Autodesk Fusion 360 part; units mm, degrees
note: some values were not read from the file. Set by a fixed rule: which face or edge a step refers to; which sketch regions a step uses.
(part 2 of 2)
sketch "Sketch3 (3)" plane through (0, 0, 1.5) normal (0, 0, -1) x (1, 0, 0) in component "fan"
  circle A0 centre (4.5, 0.1) radius 11.5
  circle A1 centre (4.5, 0.1) radius 9.5
  circle A2 centre (4.5, 0.1) radius 13
  circle A3 centre (4.5, 0.1) radius 12.5
  circle A4 centre (4.5, 0.1) radius 10 construction
  line L0 (4.5, 0.1) -> (4.5, -14.2274) construction
  arc A5 (4.6425, -10.0179) -> (4.2039, -10.2579) centre (4.4232, -10.1379) ccw
  arc A6 (5.1085, -12.3852) -> (4.6425, -10.0179) centre (1.1336, -11.9382) ccw
  arc A7 (4.603, -12.3996) -> (4.2039, -10.2579) centre (1.1336, -11.9382) ccw
  line L1 (4.5, -9.9) -> (4.35, -9.8989) construction
  arc A8 (4.4226, -12.7997) -> (4.4907, -11.4) centre (1.1336, -11.9382) ccw
  arc A9 (5.1365, -12.8252) -> (5.1953, -11.379) centre (1.1336, -11.9382) ccw
  arc A10 (5.0618, -12.8879) -> (5.1365, -12.8252) centre (5.0584, -12.8079) ccw
  arc A11 (4.4226, -12.7997) -> (4.5, -12.9) centre (4.5, -12.82) ccw
  dimension "d210" = 26
  dimension "d211" = 0.25
  dimension "d212" = 4
  dimension "d216" = 1
  dimension "d218" = 0.15
  dimension "d220" = 0.1
  dimension "d221" = 0.1
  dimension "d222" = 0.08
  constraint concentric A0 A2
  constraint concentric A2 A3
  constraint coincident A0.centre A1.centre
  constraint vertical L0
  constraint coincident A3 A6.start
  constraint tangent A5 A6
  constraint tangent A5 A7
  constraint coincident A3 A7.start
  constraint concentric A6 A7
  constraint coincident A5 L1.start
  constraint coincident A5 L1.end
  constraint coincident A4 L1.start
  constraint coincident A4 L1.end
  constraint coincident A3 A6.centre
  constraint coincident L0 L1.start
  constraint coincident A0 A8.end
  constraint coincident A0 A9.end
  constraint coincident A2 A10.start
  constraint tangent A9 A10
  constraint coincident A2 A11.end
  constraint tangent A8 A11
  constraint tangent A2 A11
  constraint tangent A2 A10
  constraint concentric A6 A9
  constraint concentric A7 A8
  constraint equal A10 A11
  measures "d210" diameter of A2
  measures "d211" radius of A5
  measures "d212" radius of A6
  measures "d216" distance of A0 A3
  measures "d218" distance of L1.start L1.end
  measures "d220" distance of A6 A9
  measures "d221" distance of A7 A8
  measures "d222" radius of A11
extrude "Extrude6''" add sketch "Sketch3 (3)" against normal up to surface (8.25 mm away) contours A0 A5 A6 A7 | A0 A3 A6 A7 picked at (4.7849, -10.7903) bodies 19 in component "fan"
extrude "Extrude7'" add sketch "Sketch3 (3)" against normal up to surface (7.5 mm away) contours A0 A3 A7 A8 | A0 A3 A6 A9 | A0 A3 A6 A7 | A2 A3 A8 A9 A10 A11 picked at (4.6466, -12.61) bodies 19 in component "fan"
pattern_circular "C-Pattern1'" count 32 over 360 about axis through (4.5, -0.1, 4.25) along (0, 0, 1) of "Extrude6''", "Extrude7'" in component "fan"
component "base" placed x (1, 0, 0) y (0, 1, 0) z (0, 0, 1) at (0, 0, 0)
component "lid" placed x (1, 0, 0) y (0, 1, 0) z (0, 0, 1) at (0, 0, 0)
component "driver and stator" placed x (1, 0, 0) y (0, 1, 0) z (0, 0, 1) at (0, 0, 0)
component "rotor" placed x (1, 0, 0) y (0, 1, 0) z (0, 0, 1) at (0, 0, 0)
component "fan" placed x (1, 0, 0) y (0, 1, 0) z (0, 0, 1) at (0, 0, 0)
equation "d28 = d13"
equation "d58 = d54"
equation "d59 = d54"
equation "d66 = d67"
equation "d68 = d67"
equation "d80 = d67"
equation "d81 = d68"
equation "d82 = d66"
equation "d116 = d115 / 2"
equation "d180 = d155"
equation "d192 = d187"
equation "d227 = 8 * 4"
